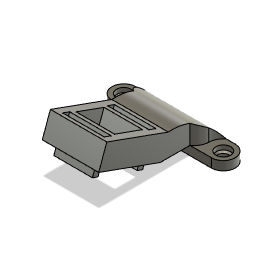
holder_v2 (Autodesk Fusion 360 design; units mm, degrees)
Autodesk Fusion 360 part; units mm, degrees
note: some values were not read from the file. Set by a fixed rule: which sketch regions a step uses.
sketch "Sketch1" plane through (0, 0, 0) normal (0, 1, 0) x (1, 0, 0)
  line L0 (0, 0) -> (33.5, 0)
  circle A0 centre (0, 0) radius 1.75
  circle A1 centre (33.5, 0) radius 1.75
  circle A2 centre (33.5, 0) radius 4
  circle A3 centre (0, 0) radius 4
  line L1 (0, 4) -> (33.5, 4)
  line L2 (33.5, -4) -> (0, -4)
  dimension "d1" = 33.5
  dimension "d2" = 3.5
  dimension "d3" = 3.5
  dimension "d4" = 8
  dimension "d5" = 8
  constraint coincident L0.start A0.centre
  constraint horizontal L0
  constraint coincident L0.end A1.centre
  constraint concentric A1 A2
  constraint coincident A3 L1.start
  constraint coincident A2 L1.end
  constraint tangent A2 L1
  constraint parallel L0 L1
  constraint coincident A2 L2.start
  constraint coincident A3 L2.end
  constraint tangent A3 L2
  constraint parallel L1 L2
  measures "d1" distance of L0.start L0.end
  measures "d2" diameter of A0
  measures "d3" diameter of A1
  measures "d4" diameter of A2
  measures "d5" diameter of A3
extrude "Extrude1" add sketch "Sketch1" along normal blind 3
hole "Hole1" at (0, 3, 0) direction (0, -1, 0) diameter 5 depth 1.5 tip angle 118
hole "Hole2" at (33.5, 3, 0) direction (0, -1, 0) diameter 5 depth 1.5 tip angle 118
sketch "Sketch2" plane through (0, 3, 0) normal (0, 1, 0) x (-1, 0, 0)
  circle A0 centre (-33.5, 0) radius 2.5
  circle A1 centre (0, 0) radius 2.5
  arc A2 (0, -4) -> (0, 4) centre (0, 0) ccw
  line L0 (0, 4) -> (-33.5, 4)
  arc A3 (-33.5, 4) -> (-33.5, -4) centre (-33.5, 0) ccw
  line L1 (-33.5, -4) -> (0, -4)
  circle A4 centre (0, 0) radius 5
  circle A5 centre (-33.5, 0) radius 5
  dimension "d16" = 10
  dimension "d17" = 10
  constraint coincident A1.centre A2.centre
  constraint concentric A0 A5
  measures "d16" diameter of A4
  measures "d17" diameter of A5
extrude "Extrude2" add sketch "Sketch2" along normal blind 10 contours L0 L1 A4 A5
sketch "Sketch3" plane through (0, 0, 0) normal (1, 0, 0) x (0, 0, -1)
  line L0 (0, 0) -> (0, 3)
  line L1 (0, 3) -> (4, 3)
  line L2 (0, 3) -> (-4, 3)
  line L3 (-4, 3) -> (-4, 13)
  arc A0 (4, 3) -> (-4, 13) centre (-6.0817, 3.1346) ccw
  line L4 (-4, 13) -> (4, 13)
  line L5 (4, 13) -> (4, 3)
  dimension "d20" = 3
  dimension "d21" = 4
  dimension "d22" = 4
  dimension "d23" = 10
  dimension "d24" = 8
  constraint coincident L0.start origin
  constraint vertical L0
  constraint perpendicular L0 L1
  constraint perpendicular L0 L2
  constraint perpendicular L2 L3
  constraint perpendicular L3 L4
  measures "d20" distance of L0.start L0.end
  measures "d21" distance of L0.end L1.end
  measures "d22" distance of L0.end L2.end
  measures "d23" distance of L2.end L3.end
  measures "d24" distance of L3.end L4.end
extrude "Extrude3" cut sketch "Sketch3" along normal blind 34.5 contours A0 L4 L5
sketch "Sketch4" plane through (0, 0, 4) normal (0, 0, 1) x (1, 0, 0)
  line L0 (0, 0) -> (33.5, 0)
  line L1 (33.5, 0) -> (33.5, 3)
  line L2 (33.5, 3) -> (30.5, 3)
  line L3 (30.5, 3) -> (30.5, 13)
  line L4 (30.5, 13) -> (3, 13)
  line L5 (3, 13) -> (3, 3)
  line L6 (3, 3) -> (0, 3)
  line L7 (0, 3) -> (0, 0)
  line L8 (3, 3) -> (30.5, 3)
  constraint coincident L5.end L6.start
  constraint coincident L2.end L3.start
extrude "Extrude4" add sketch "Sketch4" along normal blind 10 contours L3 L4 L5 L8
sketch "Sketch5" plane through (3, 0, 0) normal (-1, 0, 0) x (0, 0, 1)
  line L0 (4, 13) -> (4, 3)
  line L1 (4, 3) -> (14, 3)
  line L2 (14, 3) -> (14, 13)
  line L3 (14, 13) -> (4, 13)
  line L4 (0, 0) -> (0, -6)
  line L5 (0, -6) -> (15.5, -6)
  line L6 (15.5, -6) -> (15.5, -32)
  line L7 (15.5, -32) -> (30.5, -32)
  line L8 (30.5, -32) -> (15.5, -6)
  line L9 (14, 3) -> (34.6989, 10.4536)
  line L10 (34.6989, 10.4536) -> (31.9885, 17.9805)
  line L11 (14, 3) -> (11.2896, 10.5269)
  line L12 (11.2896, 10.5269) -> (31.9885, 17.9805)
  line L13 (14, 3) -> (-4, 3)
  arc A0 (11.2896, 10.5269) -> (-4, 3) centre (10.0878, -6.3244) ccw
  line L14 (-4, 3) -> (-4.7957, 3)
  line L15 (-4.7957, 3) -> (-4.7957, 13)
  line L16 (-4.7957, 13) -> (4, 13)
  dimension "d29" = 6
  dimension "d30" = 15.5
  dimension "d31" = 26
  dimension "d32" = 15
  dimension "d35" = 22
  dimension "d36" = 8
  dimension "d37" = 8
  dimension "d38" = 18
  constraint coincident L4.start origin
  constraint vertical L4
  constraint perpendicular L4 L5
  constraint perpendicular L5 L6
  constraint perpendicular L6 L7
  constraint coincident L1.end L2.start
  constraint perpendicular L9 L10
  constraint perpendicular L9 L11
  constraint parallel L1 L13
  constraint parallel L13 L14
  constraint perpendicular L3 L15
  constraint coincident L0.start L3.end
  constraint perpendicular L0 L16
  measures "d29" distance of L4.start L4.end
  measures "d30" distance of L4.end L5.end
  measures "d31" distance of L5.end L6.end
  measures "d32" distance of L6.end L7.end
  measures "d35" distance of L1.end L9.end
  measures "d36" distance of L9.end L10.end
  measures "d37" distance of L1.end L11.end
  measures "d38" distance of L1.end L13.end
extrude "Extrude5" cut sketch "Sketch5" against normal blind 32 contours L0 L2 L3 L12 A0 | L0 A0 L14 L15 L16
extrude "Extrude6" cut sketch "Sketch5" against normal blind 33 contours L2 L11 L12 | L2 L9 L10 L12
extrude "Extrude7" add sketch "Sketch5" against normal blind 27.5 contours L2 L11 L12 | L2 L9 L10 L12
sketch "Sketch9" plane through (0, 5.7198, -2.0597) normal (0, 0.940858, -0.3388) x (-1, 0, 0)
  line L0 (-3, 14.1884) -> (-3, 36.1884)
  line L1 (-3, 36.1884) -> (-30.5, 36.1884)
  line L2 (-30.5, 36.1884) -> (-30.5, 14.1884)
  line L3 (-30.5, 14.1884) -> (-3, 14.1884)
  line L4 (-16.75, 36.1884) -> (-16.75, 34.1884)
  line L5 (-16.75, 34.1884) -> (-16.75, 32.1884)
  line L6 (-16.75, 32.1884) -> (-16.75, 30.1884)
  line L7 (-16.75, 30.1884) -> (-16.75, 20.1884)
  line L8 (-16.75, 20.1884) -> (-16.75, 18.1884)
  line L9 (-16.75, 33.1884) -> (-16.75, 34.4384)
  line L10 (-16.75, 34.4384) -> (-9.75, 34.4384)
  line L11 (-9.75, 34.4384) -> (-23.75, 34.4384)
  line L12 (-23.75, 34.4384) -> (-23.75, 31.9384)
  line L13 (-23.75, 31.9384) -> (-9.75, 31.9384)
  line L14 (-9.75, 31.9384) -> (-9.75, 34.4384)
  line L15 (-16.75, 30.1884) -> (-10.25, 30.1884)
  line L16 (-10.25, 30.1884) -> (-23.25, 30.1884)
  line L17 (-23.25, 30.1884) -> (-23.25, 20.1884)
  line L18 (-23.25, 20.1884) -> (-10.25, 20.1884)
  line L19 (-10.25, 20.1884) -> (-10.25, 30.1884)
  line L20 (-16.75, 18.1884) -> (-16.75, 16.1884)
  line L21 (-16.75, 17.1884) -> (-16.75, 18.4384)
  line L22 (-16.75, 18.4384) -> (-9.75, 18.4384)
  line L23 (-9.75, 18.4384) -> (-23.75, 18.4384)
  line L24 (-23.75, 18.4384) -> (-23.75, 15.9384)
  line L25 (-23.75, 15.9384) -> (-9.75, 15.9384)
  line L26 (-9.75, 15.9384) -> (-9.75, 18.4384)
  dimension "d115" = 2
  dimension "d116" = 2
  dimension "d117" = 2
  dimension "d118" = 10
  dimension "d119" = 2
  dimension "d120" = 1.25
  dimension "d121" = 7
  dimension "d122" = 14
  dimension "d123" = 2.5
  dimension "d124" = 6.5
  dimension "d125" = 13
  dimension "d126" = 10
  dimension "d127" = 2
  dimension "d128" = 1.25
  dimension "d129" = 7
  dimension "d130" = 14
  dimension "d131" = 2.5
  constraint midpoint L1 L4.start
  constraint perpendicular L1 L4
  constraint vertical L5
  constraint parallel L5 L6
  constraint parallel L6 L7
  constraint parallel L7 L8
  constraint midpoint L5 L9.start
  constraint parallel L5 L9
  constraint perpendicular L9 L10
  constraint horizontal L11
  constraint vertical L12
  constraint horizontal L13
  constraint vertical L14
  constraint perpendicular L6 L15
  constraint horizontal L16
  constraint vertical L17
  constraint horizontal L18
  constraint vertical L19
  constraint parallel L8 L20
  constraint midpoint L20 L21.start
  constraint parallel L20 L21
  constraint perpendicular L21 L22
  constraint horizontal L23
  constraint vertical L24
  constraint horizontal L25
  constraint vertical L26
  measures "d115" distance of L4.start L4.end
  measures "d116" distance of L4.end L5.end
  measures "d117" distance of L5.end L6.end
  measures "d118" distance of L6.end L7.end
  measures "d119" distance of L7.end L8.end
  measures "d120" distance of L9.start L9.end
  measures "d121" distance of L9.end L10.end
  measures "d122" distance of L10.end L11.end
  measures "d123" distance of L10.end L13.end
  measures "d124" distance of L6.end L15.end
  measures "d125" distance of L15.end L16.end
  measures "d126" distance of L15.end L18.end
  measures "d127" distance of L8.end L20.end
  measures "d128" distance of L21.start L21.end
  measures "d129" distance of L21.end L22.end
  measures "d130" distance of L22.end L23.end
  measures "d131" distance of L22.end L25.end
extrude "Extrude15" cut sketch "Sketch9" against normal blind 8 contours L7 L15 L16 L18 L19 | L7 L16 L17 L18
extrude "Extrude16" cut sketch "Sketch9" against normal blind 4 contours L4 L5 L6 L9 L10 L11 L13 L14 | L4 L5 L6 L9 L11 L12 L13 | L22 L23 L24 L25 L26
sketch "Sketch10" plane through (0, -1.807, 0.6507) normal (0, -0.940858, 0.3388) x (1, 0, 0)
  line L0 (3, 36.1884) -> (3, 14.1884)
  line L1 (3, 14.1884) -> (30.5, 14.1884)
  line L2 (30.5, 14.1884) -> (30.5, 36.1884)
  line L3 (30.5, 36.1884) -> (3, 36.1884)
  line L4 (16.75, 36.1884) -> (16.75, 34.1884)
  line L5 (16.75, 34.1884) -> (23.25, 34.1884)
  line L6 (23.25, 34.1884) -> (10.25, 34.1884)
  line L7 (10.25, 34.1884) -> (10.25, 32.1884)
  line L8 (10.25, 32.1884) -> (23.25, 32.1884)
  line L9 (23.25, 32.1884) -> (23.25, 34.1884)
  line L10 (10.25, 30.1884) -> (23.25, 30.1884)
  line L11 (23.25, 30.1884) -> (23.25, 20.1884)
  line L12 (23.25, 20.1884) -> (10.25, 20.1884)
  line L13 (10.25, 20.1884) -> (10.25, 30.1884)
  line L14 (16.75, 32.1884) -> (16.75, 18.1884)
  line L15 (16.75, 18.1884) -> (23.25, 18.1884)
  line L16 (23.25, 18.1884) -> (10.25, 18.1884)
  line L17 (10.25, 18.1884) -> (10.25, 16.1884)
  line L18 (10.25, 16.1884) -> (23.25, 16.1884)
  line L19 (23.25, 16.1884) -> (23.25, 18.1884)
  dimension "d111" = 2
  dimension "d112" = 6.5
  dimension "d113" = 13
  dimension "d114" = 2
  dimension "d132" = 14
  dimension "d133" = 6.5
  dimension "d134" = 13
  dimension "d135" = 2
  constraint midpoint L3 L4.start
  constraint perpendicular L3 L4
  constraint perpendicular L4 L5
  constraint horizontal L6
  constraint vertical L7
  constraint horizontal L8
  constraint vertical L9
  constraint midpoint L8 L14.start
  constraint perpendicular L12 L14
  constraint perpendicular L14 L15
  constraint horizontal L16
  constraint vertical L17
  constraint horizontal L18
  constraint vertical L19
  measures "d111" distance of L4.start L4.end
  measures "d112" distance of L4.end L5.end
  measures "d113" distance of L5.end L6.end
  measures "d114" distance of L5.end L8.end
  measures "d132" distance of L14.start L14.end
  measures "d133" distance of L14.end L15.end
  measures "d134" distance of L15.end L16.end
  measures "d135" distance of L15.end L18.end
extrude "Extrude17" add sketch "Sketch10" along normal blind 3 contours L5 L6 L7 L8 L9 | L15 L16 L17 L18 L19
extrude "Extrude18" cut 1 faces at (3, 7.9935, 19.9962) along direction (1, 0, 0) blind 4.25
extrude "Extrude19" cut 1 faces at (30.5, 10.5024, 19.0927) along direction (-1, 0, 0) blind 4.25
fillet "Fillet1" radius 5 2 edges at (3, 6.2173, 4) (30.5, 6.2173, 4)
equation "d112 = ( 13 / 2 ) * 1 mm"
equation "d120 = ( 2.5 / 2 ) * 1 mm"
equation "d124 = ( 13 / 2 ) * 1 mm"
equation "d128 = ( 2.5 / 2 ) * 1 mm"
